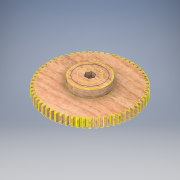
# Autodesk Inventor part: gear2
Saved by Autodesk Inventor 2018 (Build 220112000, 112)
## iProperties
Created: 2019-02-16
Part Number: gear2
Material: Generic
Description: SolidWorks IGES file using analytic representation for surfaces
Document SubType Name: Modeling
Designer: snipe
Density: 1 g/cm^3
Appearance: Default
Sending System: SolidWorks 2018
Preprocessor: SolidWorks 2018
Minimum Resolution: 0.0
Sending System Product ID: 48_gear2
Receiving System Product ID: 48_gear2
Sent Units: Millimeter
Translation Standard: IGES 5.3
Model Creation Time: 2019-02-16
Title: C:\Users\Admin\Desktop\48_gear2.IGS
Author: Admin
Autodesk Inventor part; units mm, degrees
ref_plane "YZ Plane" through (0, 0, 0) normal (1, 0, 0) x (0, 1, 0)
ref_plane "XZ Plane" through (0, 0, 0) normal (0, 1, 0) x (-1, 0, 0)
ref_plane "XY Plane" through (0, 0, 0) normal (0, 0, 1) x (1, 0, 0)
surface "Composite1"
sketch "Sketch1" plane through (0, 19, 0) normal (0, 1, 0) x (1, 0, 0)
  line L0 (6.35, 0) -> (3.175, -5.4993)
  line L1 (3.175, -5.4993) -> (-3.175, -5.4993)
  line L2 (-3.175, -5.4993) -> (-6.35, 0)
  line L3 (-6.35, 0) -> (-3.175, 5.4993)
  line L4 (-3.175, 5.4993) -> (3.175, 5.4993)
  line L5 (3.175, 5.4993) -> (6.35, 0)
  circle A0 centre (0, 0) radius 20
  dimension "d0" = 12.7
  dimension "d1" = 40
  constraints: 12 end point, 2 coincident, 1 centre point, 13 other
  measures "d0" distance of L0.start L2.end
  measures "d1" diameter of A0
extrude "Extrusion1" add sketch "Sketch1" against normal up to surface (38 mm away)
body "Solid1"
body "Srf1"
